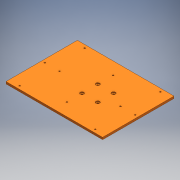
# Autodesk Inventor part: widefieldViewingPlatformBase
Saved by Autodesk Inventor 2016 (Build 200138000, 138)
## iProperties
Created: 2016-03-18
Part Number: widefieldViewingPlatformBase
Material: Generic
Document SubType Name: Modeling
Designer: sims01
Density: 1 g/cm^3
Appearance: Default
Author: sims01
Autodesk Inventor part; units mm, degrees
ref_plane "YZ Plane" through (0, 0, 0) normal (1, 0, 0) x (0, 1, 0)
ref_plane "XZ Plane" through (0, 0, 0) normal (0, 1, 0) x (-1, 0, 0)
ref_plane "XY Plane" through (0, 0, 0) normal (0, 0, 1) x (1, 0, 0)
sketch "Sketch1" plane through (0, 0, 0) normal (0, 0, 1) x (1, 0, 0)
  line L0 (-85.05, 54.7) -> (85.05, 54.7)
  line L1 (85.05, 54.7) -> (85.05, -54.7)
  line L2 (85.05, -54.7) -> (-85.05, -54.7)
  line L3 (-85.05, -54.7) -> (-85.05, 54.7)
  point P0 (0, 0)
  dimension "d0" = 170.1
  dimension "d1" = 85.05
  dimension "d2" = 109.4
  dimension "d3" = 54.7
  constraints: 8 end point, 2 parallel, 1 horizontal, 1 perpendicular
  measures "d0" distance of L0.start L0.end
  measures "d1" distance from line of point (0, 0) L1
  measures "d2" distance of L0.end L1.end
  measures "d3" distance from line of point (0, 0) L0
extrude "baseExtrusion" add sketch "Sketch1" along normal blind 10
sketch "Sketch2" plane through (0, 0, 10) normal (0, 0, 1) x (1, 0, 0)
  line L0 (85.05, -54.7) -> (85.05, 54.7) projected
  point P0 (0, 0)
  point P1 (-0.55, 37.5)
  point P2 (-0.55, -37.5)
  point P3 (74.45, 37.5)
  point P4 (74.45, -37.5)
  dimension "d6" = 75
  dimension "d7" = 75
  dimension "d9" = 37.5
  dimension "d17" = 10.6
  constraints: 2 horizontal alignment, 2 vertical alignment
  measures "d6" distance of point (-0.55, 37.5) point (74.45, 37.5)
  measures "d7" distance of point (74.45, -37.5) point (74.45, 37.5)
  measures "d9" vertical distance of point (0, 0) point (74.45, 37.5)
  measures "d17" distance from line of L0 point (74.45, 37.5)
hole "zStageM6MountingHoles" at (-0.55, 37.5, 10) at (-0.55, -37.5, 10) at (74.45, 37.5, 10) at (74.45, -37.5, 10) direction (0, 0, -1) diameter 6.6 end through all counterbore diameter 18 counterbore depth 4.8 clearance for "Hex Head Cap Screw ISO 24017" size "M6" standard "ISO"
sketch "Sketch5" plane through (0, 0, 10) normal (0, 0, 1) x (1, 0, 0)
  line L0 (230, -170) -> (-230, -170)
  line L1 (-230, -170) -> (-230, 170)
  line L2 (-230, 170) -> (230, 170)
  line L3 (230, 170) -> (230, -170)
  line L4 (-85.05, -54.7) -> (85.05, -54.7) projected
  line L5 (85.05, 54.7) -> (-85.05, 54.7) projected
  line L6 (85.05, -54.7) -> (85.05, 54.7) projected
  line L7 (-85.05, 54.7) -> (-85.05, -54.7) projected
  point P0 (0, 0)
  dimension "d44" = 340
  dimension "d45" = 170
  dimension "d46" = 460
  dimension "d47" = 230
  constraints: 8 end point, 2 parallel, 1 horizontal, 1 perpendicular
  measures "d44" distance of L2.end L0.start
  measures "d45" distance from line of point (0, 0) L0
  measures "d46" distance of L0.start L0.end
  measures "d47" distance from line of point (0, 0) L3
extrude "excessExtrusion" add sketch "Sketch5" against normal blind 10
sketch "Sketch7" plane through (0, 0, 0) normal (0, 0, -1) x (-1, 0, 0)
  line L0 (230, -170) -> (230, 170) projected
  line L1 (230, 170) -> (-230, 170) projected
  line L2 (-230, -170) -> (230, -170) projected
  point P0 (0, 0)
  point P1 (180, -155)
  point P2 (215, 0)
  point P3 (145, 0)
  point P4 (0, -110)
  dimension "d48" = 15
  dimension "d50" = 15
  dimension "d51" = 85
  dimension "d60" = 50
  dimension "d61" = 60
  constraints: 2 horizontal alignment, 1 vertical alignment
  measures "d48" distance from line of L0 point (215, 0)
  measures "d50" distance from line of L2 point (180, -155)
  measures "d51" distance from line of L0 point (145, 0)
  measures "d60" distance from line of L0 point (180, -155)
  measures "d61" distance from line of L2 point (0, -110)
hole "Hole4" at (-180, -155, 0) at (-215, 0, 0) at (-145, 0, 0) at (0, -110, 0) direction (0, 0, 1) diameter 6.6 end through all counterbore diameter 18 counterbore depth 4.8 clearance for "Hex Head Cap Screw ISO 24017" size "M6" standard "ISO"
mirror "Mirror7" about plane through (0, 0, 0) normal (1, 0, 0) of "Hole4"
mirror "Mirror8" about plane through (0, 0, 0) normal (0, 1, 0) of "Hole4", "Mirror7"
equation "\"d1\" = 0.5 * d0"
equation "\"d3\" = 0.5 * d2"
equation "\"d9\" = 0.5 * d7"
equation "\"d45\" = 0.5 * d44"
equation "\"d47\" = 0.5 * d46"
body "Solid1"
